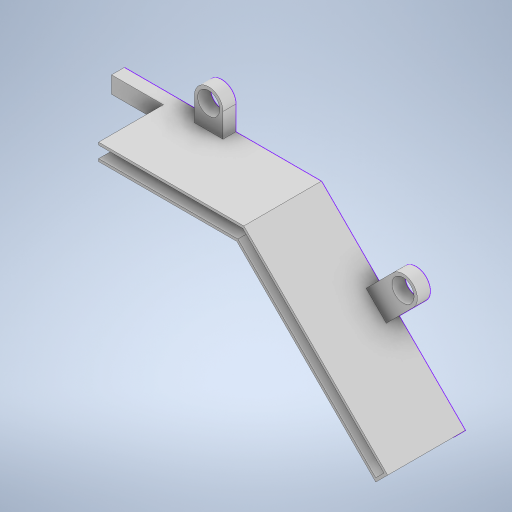
# Autodesk Inventor part: hold_right_sim
Saved by Autodesk Inventor 2024 (Build 280153000, 153)
## iProperties
Created: 2024-02-27
Part Number: hold_right_sim
Material: Generic
Document SubType Name: Modeling
Designer: Administrator
Density: 1 g/cm^3
Appearance: Default
Author: Administrator
Autodesk Inventor part; units mm, degrees
ref_plane "YZ Plane" through (0, 0, 0) normal (1, 0, 0) x (0, 1, 0)
ref_plane "XZ Plane" through (0, 0, 0) normal (0, 1, 0) x (-1, 0, 0)
ref_plane "XY Plane" through (0, 0, 0) normal (0, 0, 1) x (1, 0, 0)
sketch "Sketch1" plane through (0, 0, 0) normal (0, 0, 1) x (1, 0, 0)
  line L0 (0.1713, 1.5278) -> (0.1713, -1.4722)
  line L1 (0.1713, 1.5278) -> (0.1713, 6.5278)
  line L2 (0.1713, -1.4722) -> (0.1713, -6.4722)
  line L3 (0.1713, -6.4722) -> (146.8575, -6.4722)
  line L4 (152.2423, 6.5278) -> (0.1713, 6.5278)
  line L5 (146.8575, -6.4722) -> (254.1159, -113.7306)
  line L6 (263.3083, -104.5382) -> (152.2423, 6.5278)
  line L7 (254.1159, -113.7306) -> (263.3083, -104.5382)
  line L8 (40.1713, -6.4722) -> (40.1713, -4.4722)
  line L9 (232.9494, -32.7504) -> (212.235, -53.4648)
  circle A0 centre (225.1713, -24.9722) radius 8.5
  circle A1 centre (225.1713, -24.9722) radius 11
  line L10 (217.3931, -17.194) -> (196.6786, -37.9085)
  line L11 (182.9494, -82.7504) -> (203.0426, -62.6572)
  line L12 (167.3931, -67.194) -> (187.4862, -47.1009)
  circle A2 centre (175.1713, -74.9722) radius 8.5
  circle A3 centre (175.1713, -74.9722) radius 11
  line L13 (86.1713, -24.9722) -> (86.1713, -6.4722)
  line L14 (64.1713, -24.9722) -> (64.1713, -6.4722)
  circle A4 centre (75.1713, -24.9722) radius 8.5
  circle A5 centre (75.1713, -24.9722) radius 11
  line L15 (86.1713, 25.0278) -> (86.1713, 6.5278)
  circle A6 centre (75.1713, 25.0278) radius 8.5
  circle A7 centre (75.1713, 25.0278) radius 11
  line L16 (64.1713, 25.0278) -> (64.1713, 6.5278)
  line L17 (40.1713, 4.5278) -> (40.1713, 6.5278)
  line L18 (40.1713, 4.5278) -> (151.4139, 4.5278)
  line L19 (151.4139, 4.5278) -> (260.4799, -104.5382)
  line L20 (260.4799, -104.5382) -> (254.1159, -110.9022)
  line L21 (254.1159, -110.9022) -> (147.686, -4.4722)
  line L22 (147.686, -4.4722) -> (40.1713, -4.4722)
  point P0 (0, 0)
  point P1 (0.1713, 0.0278)
  point P2 (0.1713, 0.0278)
  point P3 (0.1713, -3.9722)
  point P4 (40.1713, -3.9722)
  point P5 (76.2068, 6.5278)
  point P6 (86.1713, 6.5278)
  point P7 (64.1713, 6.5278)
  point P8 (86.1713, -6.4722)
  point P9 (64.1713, -6.4722)
  point P10 (203.0426, -62.6572)
  point P11 (187.4862, -47.1009)
  point P12 (196.6786, -37.9085)
  point P13 (212.235, -53.4648)
  constraints: 46 end point, 8 centre point, 8 point on circle, 4 coincident, 4 point on line, 2 midpoint, 1 perpendicular, 1 tangent
extrude "Extrusion4" add sketch "Sketch1" along normal blind 60 contours L4 L6 L7 L5 L3 L8 L22 L21 L20 L19 L18 L17
extrude "Extrusion5" add sketch "Sketch1" along normal blind 10 contours L1 L4 L17 L18 L19 L20 L21 L22 L8 L3 L2 L0 | L16 A7 L15 L4 | L3 L13 A5 L14 | A7 | A5 | L10 A1 L9 L6 | L5 L11 A3 L12 | A1 | A3
body "Solid2"
